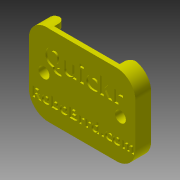
# Autodesk Inventor part: quickr_v1
Saved by Autodesk Inventor 2014 SP1 (Build 180222100, 222)
## iProperties
Created: 2014-02-28
Part Number: quickr_v1
Material: Generic
Document SubType Name: Modeling
Designer: Erin
Density: 1 g/cm^3
Appearance: Default
Author: Erin
Autodesk Inventor part; units mm, degrees
(part 1 of 3)
ref_plane "YZ Plane" through (0, 0, 0) normal (1, 0, 0) x (0, 1, 0)
ref_plane "XY Plane" through (0, 0, 0) normal (0, 0, 1) x (1, 0, 0)
sketch "Sketch1" plane through (0, 0, 0) normal (0, 1, 0) x (-1, 0, 0)
  line L0 (29.241, 31.084) -> (29.241, 17.6221)
  line L1 (0.285, 31.084) -> (0.285, 17.368)
  line L2 (4.095, 13.8121) -> (25.431, 13.8121)
  spline S0 degree 3 poles (29.241, 17.6221) (29.241, 15.518) (27.5351, 13.8121) (25.431, 13.8121) knots 0 0 0 0 1 1 1 1
  line L3 (29.241, 17.6221) -> (29.241, 15.518) construction
  line L4 (29.241, 15.518) -> (27.5351, 13.8121) construction
  line L5 (27.5351, 13.8121) -> (25.431, 13.8121) construction
  spline S1 degree 3 poles (4.095, 13.8121) (1.9909, 13.8121) (0.285, 15.518) (0.285, 17.6221) knots 0 0 0 0 1 1 1 1
  line L6 (4.095, 13.8121) -> (1.9909, 13.8121) construction
  line L7 (1.9909, 13.8121) -> (0.285, 15.518) construction
  line L8 (0.285, 15.518) -> (0.285, 17.6221) construction
  spline S2 degree 3 poles (25.431, 34.64) (27.5351, 34.64) (29.241, 32.9341) (29.241, 30.83) knots 0 0 0 0 1 1 1 1
  line L9 (25.431, 34.64) -> (27.5351, 34.64) construction
  line L10 (27.5351, 34.64) -> (29.241, 32.9341) construction
  line L11 (29.241, 32.9341) -> (29.241, 30.83) construction
  spline S3 degree 3 poles (0.285, 30.83) (0.285, 32.9341) (1.9909, 34.64) (4.095, 34.64) knots 0 0 0 0 1 1 1 1
  line L12 (0.285, 30.83) -> (0.285, 32.9341) construction
  line L13 (0.285, 32.9341) -> (1.9909, 34.64) construction
  line L14 (1.9909, 34.64) -> (4.095, 34.64) construction
  line L15 (25.431, 34.64) -> (3.841, 34.64)
  line L16 (10.9529, 29.56) -> (10.9529, 29.3061)
  spline S4 degree 3 poles (14.4582, 19.1461) (14.4582, 19.6791) (14.026, 20.1112) (13.4929, 20.1112) knots 0 0 0 0 1 1 1 1
  line L17 (14.4582, 19.1461) -> (14.4582, 19.6791) construction
  line L18 (14.4582, 19.6791) -> (14.026, 20.1112) construction
  line L19 (14.026, 20.1112) -> (13.4929, 20.1112) construction
  spline S5 degree 3 poles (13.4929, 20.1112) (12.9599, 20.1112) (12.5277, 19.6791) (12.5277, 19.1461) knots 0 0 0 0 1 1 1 1
  line L20 (13.4929, 20.1112) -> (12.9599, 20.1112) construction
  line L21 (12.9599, 20.1112) -> (12.5277, 19.6791) construction
  line L22 (12.5277, 19.6791) -> (12.5277, 19.1461) construction
  spline S6 degree 3 poles (12.5277, 19.1461) (12.5277, 18.613) (12.9599, 18.1809) (13.4929, 18.1809) knots 0 0 0 0 1 1 1 1
  line L23 (12.5277, 19.1461) -> (12.5277, 18.613) construction
  line L24 (12.5277, 18.613) -> (12.9599, 18.1809) construction
  line L25 (12.9599, 18.1809) -> (13.4929, 18.1809) construction
  spline S7 degree 3 poles (13.4929, 18.1809) (14.026, 18.1809) (14.4582, 18.613) (14.4582, 19.1461) knots 0 0 0 0 1 1 1 1
  line L26 (13.4929, 18.1809) -> (14.026, 18.1809) construction
  line L27 (14.026, 18.1809) -> (14.4582, 18.613) construction
  line L28 (14.4582, 18.613) -> (14.4582, 19.1461) construction
  spline S8 degree 3 poles (16.9982, 19.1461) (16.9982, 19.6791) (16.566, 20.1112) (16.0329, 20.1112) knots 0 0 0 0 1 1 1 1
  line L29 (16.9982, 19.1461) -> (16.9982, 19.6791) construction
  line L30 (16.9982, 19.6791) -> (16.566, 20.1112) construction
  line L31 (16.566, 20.1112) -> (16.0329, 20.1112) construction
  spline S9 degree 3 poles (16.0329, 20.1112) (15.4999, 20.1112) (15.0677, 19.6791) (15.0677, 19.1461) knots 0 0 0 0 1 1 1 1
  line L32 (16.0329, 20.1112) -> (15.4999, 20.1112) construction
  line L33 (15.4999, 20.1112) -> (15.0677, 19.6791) construction
  line L34 (15.0677, 19.6791) -> (15.0677, 19.1461) construction
  spline S10 degree 3 poles (15.0677, 19.1461) (15.0677, 18.613) (15.4999, 18.1809) (16.0329, 18.1809) knots 0 0 0 0 1 1 1 1
  line L35 (15.0677, 19.1461) -> (15.0677, 18.613) construction
  line L36 (15.0677, 18.613) -> (15.4999, 18.1809) construction
  line L37 (15.4999, 18.1809) -> (16.0329, 18.1809) construction
  spline S11 degree 3 poles (16.0329, 18.1809) (16.566, 18.1809) (16.9982, 18.613) (16.9982, 19.1461) knots 0 0 0 0 1 1 1 1
  line L38 (16.0329, 18.1809) -> (16.566, 18.1809) construction
  line L39 (16.566, 18.1809) -> (16.9982, 18.613) construction
  line L40 (16.9982, 18.613) -> (16.9982, 19.1461) construction
  spline S12 degree 3 poles (11.9182, 19.1461) (11.9182, 19.6791) (11.486, 20.1112) (10.9529, 20.1112) knots 0 0 0 0 1 1 1 1
  line L41 (11.9182, 19.1461) -> (11.9182, 19.6791) construction
  line L42 (11.9182, 19.6791) -> (11.486, 20.1112) construction
  line L43 (11.486, 20.1112) -> (10.9529, 20.1112) construction
  spline S13 degree 3 poles (10.9529, 20.1112) (10.4199, 20.1112) (9.9877, 19.6791) (9.9877, 19.1461) knots 0 0 0 0 1 1 1 1
  line L44 (10.9529, 20.1112) -> (10.4199, 20.1112) construction
  line L45 (10.4199, 20.1112) -> (9.9877, 19.6791) construction
  line L46 (9.9877, 19.6791) -> (9.9877, 19.1461) construction
  spline S14 degree 3 poles (9.9877, 19.1461) (9.9877, 18.613) (10.4199, 18.1809) (10.9529, 18.1809) knots 0 0 0 0 1 1 1 1
  line L47 (9.9877, 19.1461) -> (9.9877, 18.613) construction
  line L48 (9.9877, 18.613) -> (10.4199, 18.1809) construction
  line L49 (10.4199, 18.1809) -> (10.9529, 18.1809) construction
  spline S15 degree 3 poles (10.9529, 18.1809) (11.486, 18.1809) (11.9182, 18.613) (11.9182, 19.1461) knots 0 0 0 0 1 1 1 1
  line L50 (10.9529, 18.1809) -> (11.486, 18.1809) construction
  line L51 (11.486, 18.1809) -> (11.9182, 18.613) construction
  line L52 (11.9182, 18.613) -> (11.9182, 19.1461) construction
  spline S16 degree 3 poles (9.3782, 19.1461) (9.3782, 19.6791) (8.946, 20.1112) (8.4129, 20.1112) knots 0 0 0 0 1 1 1 1
  line L53 (9.3782, 19.1461) -> (9.3782, 19.6791) construction
  line L54 (9.3782, 19.6791) -> (8.946, 20.1112) construction
  line L55 (8.946, 20.1112) -> (8.4129, 20.1112) construction
  spline S17 degree 3 poles (8.4129, 20.1112) (7.8799, 20.1112) (7.4477, 19.6791) (7.4477, 19.1461) knots 0 0 0 0 1 1 1 1
  line L56 (8.4129, 20.1112) -> (7.8799, 20.1112) construction
  line L57 (7.8799, 20.1112) -> (7.4477, 19.6791) construction
  line L58 (7.4477, 19.6791) -> (7.4477, 19.1461) construction
  spline S18 degree 3 poles (7.4477, 19.1461) (7.4477, 18.613) (7.8799, 18.1809) (8.4129, 18.1809) knots 0 0 0 0 1 1 1 1
  line L59 (7.4477, 19.1461) -> (7.4477, 18.613) construction
  line L60 (7.4477, 18.613) -> (7.8799, 18.1809) construction
  line L61 (7.8799, 18.1809) -> (8.4129, 18.1809) construction
  spline S19 degree 3 poles (8.4129, 18.1809) (8.946, 18.1809) (9.3782, 18.613) (9.3782, 19.1461) knots 0 0 0 0 1 1 1 1
  line L62 (8.4129, 18.1809) -> (8.946, 18.1809) construction
  line L63 (8.946, 18.1809) -> (9.3782, 18.613) construction
  line L64 (9.3782, 18.613) -> (9.3782, 19.1461) construction
  spline S20 degree 3 poles (6.8382, 19.1461) (6.8382, 19.6791) (6.406, 20.1112) (5.8729, 20.1112) knots 0 0 0 0 1 1 1 1
  line L65 (6.8382, 19.1461) -> (6.8382, 19.6791) construction
  line L66 (6.8382, 19.6791) -> (6.406, 20.1112) construction
  line L67 (6.406, 20.1112) -> (5.8729, 20.1112) construction
  spline S21 degree 3 poles (5.8729, 20.1112) (5.3399, 20.1112) (4.9077, 19.6791) (4.9077, 19.1461) knots 0 0 0 0 1 1 1 1
  line L68 (5.8729, 20.1112) -> (5.3399, 20.1112) construction
  line L69 (5.3399, 20.1112) -> (4.9077, 19.6791) construction
  line L70 (4.9077, 19.6791) -> (4.9077, 19.1461) construction
  spline S22 degree 3 poles (4.9077, 19.1461) (4.9077, 18.613) (5.3399, 18.1809) (5.8729, 18.1809) knots 0 0 0 0 1 1 1 1
  line L71 (4.9077, 19.1461) -> (4.9077, 18.613) construction
  line L72 (4.9077, 18.613) -> (5.3399, 18.1809) construction
  line L73 (5.3399, 18.1809) -> (5.8729, 18.1809) construction
  spline S23 degree 3 poles (5.8729, 18.1809) (6.406, 18.1809) (6.8382, 18.613) (6.8382, 19.1461) knots 0 0 0 0 1 1 1 1
  line L74 (5.8729, 18.1809) -> (6.406, 18.1809) construction
  line L75 (6.406, 18.1809) -> (6.8382, 18.613) construction
  line L76 (6.8382, 18.613) -> (6.8382, 19.1461) construction
  spline S24 degree 3 poles (6.8382, 15.3361) (6.8382, 15.8691) (6.406, 16.3012) (5.8729, 16.3012) knots 0 0 0 0 1 1 1 1
  line L77 (6.8382, 15.3361) -> (6.8382, 15.8691) construction
  line L78 (6.8382, 15.8691) -> (6.406, 16.3012) construction
  line L79 (6.406, 16.3012) -> (5.8729, 16.3012) construction
  spline S25 degree 3 poles (5.8729, 16.3012) (5.3399, 16.3012) (4.9077, 15.8691) (4.9077, 15.3361) knots 0 0 0 0 1 1 1 1
  line L80 (5.8729, 16.3012) -> (5.3399, 16.3012) construction
  line L81 (5.3399, 16.3012) -> (4.9077, 15.8691) construction
  line L82 (4.9077, 15.8691) -> (4.9077, 15.3361) construction
  spline S26 degree 3 poles (4.9077, 15.3361) (4.9077, 14.803) (5.3399, 14.3709) (5.8729, 14.3709) knots 0 0 0 0 1 1 1 1
  line L83 (4.9077, 15.3361) -> (4.9077, 14.803) construction
  line L84 (4.9077, 14.803) -> (5.3399, 14.3709) construction
  line L85 (5.3399, 14.3709) -> (5.8729, 14.3709) construction
  spline S27 degree 3 poles (5.8729, 14.3709) (6.406, 14.3709) (6.8382, 14.803) (6.8382, 15.3361) knots 0 0 0 0 1 1 1 1
  line L86 (5.8729, 14.3709) -> (6.406, 14.3709) construction
  line L87 (6.406, 14.3709) -> (6.8382, 14.803) construction
  line L88 (6.8382, 14.803) -> (6.8382, 15.3361) construction
  spline S28 degree 3 poles (9.3782, 15.3361) (9.3782, 15.8691) (8.946, 16.3012) (8.4129, 16.3012) knots 0 0 0 0 1 1 1 1
  line L89 (9.3782, 15.3361) -> (9.3782, 15.8691) construction
  line L90 (9.3782, 15.8691) -> (8.946, 16.3012) construction
  line L91 (8.946, 16.3012) -> (8.4129, 16.3012) construction
  spline S29 degree 3 poles (8.4129, 16.3012) (7.8799, 16.3012) (7.4477, 15.8691) (7.4477, 15.3361) knots 0 0 0 0 1 1 1 1
  line L92 (8.4129, 16.3012) -> (7.8799, 16.3012) construction
  line L93 (7.8799, 16.3012) -> (7.4477, 15.8691) construction
  line L94 (7.4477, 15.8691) -> (7.4477, 15.3361) construction
  spline S30 degree 3 poles (7.4477, 15.3361) (7.4477, 14.803) (7.8799, 14.3709) (8.4129, 14.3709) knots 0 0 0 0 1 1 1 1
  line L95 (7.4477, 15.3361) -> (7.4477, 14.803) construction
  line L96 (7.4477, 14.803) -> (7.8799, 14.3709) construction
  line L97 (7.8799, 14.3709) -> (8.4129, 14.3709) construction
  spline S31 degree 3 poles (8.4129, 14.3709) (8.946, 14.3709) (9.3782, 14.803) (9.3782, 15.3361) knots 0 0 0 0 1 1 1 1
  line L98 (8.4129, 14.3709) -> (8.946, 14.3709) construction
  line L99 (8.946, 14.3709) -> (9.3782, 14.803) construction
  line L100 (9.3782, 14.803) -> (9.3782, 15.3361) construction
  spline S32 degree 3 poles (19.5382, 19.1461) (19.5382, 19.6791) (19.106, 20.1112) (18.5729, 20.1112) knots 0 0 0 0 1 1 1 1
  line L101 (19.5382, 19.1461) -> (19.5382, 19.6791) construction
  line L102 (19.5382, 19.6791) -> (19.106, 20.1112) construction
  line L103 (19.106, 20.1112) -> (18.5729, 20.1112) construction
  spline S33 degree 3 poles (18.5729, 20.1112) (18.0399, 20.1112) (17.6077, 19.6791) (17.6077, 19.1461) knots 0 0 0 0 1 1 1 1
  line L104 (18.5729, 20.1112) -> (18.0399, 20.1112) construction
  line L105 (18.0399, 20.1112) -> (17.6077, 19.6791) construction
  line L106 (17.6077, 19.6791) -> (17.6077, 19.1461) construction
  spline S34 degree 3 poles (17.6077, 19.1461) (17.6077, 18.613) (18.0399, 18.1809) (18.5729, 18.1809) knots 0 0 0 0 1 1 1 1
  line L107 (17.6077, 19.1461) -> (17.6077, 18.613) construction
  line L108 (17.6077, 18.613) -> (18.0399, 18.1809) construction
  line L109 (18.0399, 18.1809) -> (18.5729, 18.1809) construction
  spline S35 degree 3 poles (18.5729, 18.1809) (19.106, 18.1809) (19.5382, 18.613) (19.5382, 19.1461) knots 0 0 0 0 1 1 1 1
  line L110 (18.5729, 18.1809) -> (19.106, 18.1809) construction
  line L111 (19.106, 18.1809) -> (19.5382, 18.613) construction
  line L112 (19.5382, 18.613) -> (19.5382, 19.1461) construction
  spline S36 degree 3 poles (22.0782, 19.1461) (22.0782, 19.6791) (21.646, 20.1112) (21.1129, 20.1112) knots 0 0 0 0 1 1 1 1
  line L113 (22.0782, 19.1461) -> (22.0782, 19.6791) construction
  line L114 (22.0782, 19.6791) -> (21.646, 20.1112) construction
  line L115 (21.646, 20.1112) -> (21.1129, 20.1112) construction
  spline S37 degree 3 poles (21.1129, 20.1112) (20.5799, 20.1112) (20.1477, 19.6791) (20.1477, 19.1461) knots 0 0 0 0 1 1 1 1
  line L116 (21.1129, 20.1112) -> (20.5799, 20.1112) construction
  line L117 (20.5799, 20.1112) -> (20.1477, 19.6791) construction
  line L118 (20.1477, 19.6791) -> (20.1477, 19.1461) construction
  spline S38 degree 3 poles (20.1477, 19.1461) (20.1477, 18.613) (20.5799, 18.1809) (21.1129, 18.1809) knots 0 0 0 0 1 1 1 1
  line L119 (20.1477, 19.1461) -> (20.1477, 18.613) construction
  line L120 (20.1477, 18.613) -> (20.5799, 18.1809) construction
  line L121 (20.5799, 18.1809) -> (21.1129, 18.1809) construction
  spline S39 degree 3 poles (21.1129, 18.1809) (21.646, 18.1809) (22.0782, 18.613) (22.0782, 19.1461) knots 0 0 0 0 1 1 1 1
  line L122 (21.1129, 18.1809) -> (21.646, 18.1809) construction
  line L123 (21.646, 18.1809) -> (22.0782, 18.613) construction
  line L124 (22.0782, 18.613) -> (22.0782, 19.1461) construction
  spline S40 degree 3 poles (24.6182, 19.1461) (24.6182, 19.6791) (24.186, 20.1112) (23.6529, 20.1112) knots 0 0 0 0 1 1 1 1
  line L125 (24.6182, 19.1461) -> (24.6182, 19.6791) construction
  line L126 (24.6182, 19.6791) -> (24.186, 20.1112) construction
  line L127 (24.186, 20.1112) -> (23.6529, 20.1112) construction
  spline S41 degree 3 poles (23.6529, 20.1112) (23.1199, 20.1112) (22.6877, 19.6791) (22.6877, 19.1461) knots 0 0 0 0 1 1 1 1
  line L128 (23.6529, 20.1112) -> (23.1199, 20.1112) construction
  line L129 (23.1199, 20.1112) -> (22.6877, 19.6791) construction
  line L130 (22.6877, 19.6791) -> (22.6877, 19.1461) construction
  spline S42 degree 3 poles (22.6877, 19.1461) (22.6877, 18.613) (23.1199, 18.1809) (23.6529, 18.1809) knots 0 0 0 0 1 1 1 1
  line L131 (22.6877, 19.1461) -> (22.6877, 18.613) construction
  line L132 (22.6877, 18.613) -> (23.1199, 18.1809) construction
  line L133 (23.1199, 18.1809) -> (23.6529, 18.1809) construction
  spline S43 degree 3 poles (23.6529, 18.1809) (24.186, 18.1809) (24.6182, 18.613) (24.6182, 19.1461) knots 0 0 0 0 1 1 1 1
  line L134 (23.6529, 18.1809) -> (24.186, 18.1809) construction
  line L135 (24.186, 18.1809) -> (24.6182, 18.613) construction
  line L136 (24.6182, 18.613) -> (24.6182, 19.1461) construction
  spline S44 degree 3 poles (11.9182, 15.3361) (11.9182, 15.8691) (11.486, 16.3012) (10.9529, 16.3012) knots 0 0 0 0 1 1 1 1
  line L137 (11.9182, 15.3361) -> (11.9182, 15.8691) construction
  line L138 (11.9182, 15.8691) -> (11.486, 16.3012) construction
  line L139 (11.486, 16.3012) -> (10.9529, 16.3012) construction
  spline S45 degree 3 poles (10.9529, 16.3012) (10.4199, 16.3012) (9.9877, 15.8691) (9.9877, 15.3361) knots 0 0 0 0 1 1 1 1
  line L140 (10.9529, 16.3012) -> (10.4199, 16.3012) construction
  line L141 (10.4199, 16.3012) -> (9.9877, 15.8691) construction
  line L142 (9.9877, 15.8691) -> (9.9877, 15.3361) construction
  spline S46 degree 3 poles (9.9877, 15.3361) (9.9877, 14.803) (10.4199, 14.3709) (10.9529, 14.3709) knots 0 0 0 0 1 1 1 1
  line L143 (9.9877, 15.3361) -> (9.9877, 14.803) construction
  line L144 (9.9877, 14.803) -> (10.4199, 14.3709) construction
  line L145 (10.4199, 14.3709) -> (10.9529, 14.3709) construction
  spline S47 degree 3 poles (10.9529, 14.3709) (11.486, 14.3709) (11.9182, 14.803) (11.9182, 15.3361) knots 0 0 0 0 1 1 1 1
  line L146 (10.9529, 14.3709) -> (11.486, 14.3709) construction
  line L147 (11.486, 14.3709) -> (11.9182, 14.803) construction
  line L148 (11.9182, 14.803) -> (11.9182, 15.3361) construction
  spline S48 degree 3 poles (14.4582, 15.3361) (14.4582, 15.8691) (14.026, 16.3012) (13.4929, 16.3012) knots 0 0 0 0 1 1 1 1
  line L149 (14.4582, 15.3361) -> (14.4582, 15.8691) construction
  line L150 (14.4582, 15.8691) -> (14.026, 16.3012) construction
  line L151 (14.026, 16.3012) -> (13.4929, 16.3012) construction
  spline S49 degree 3 poles (13.4929, 16.3012) (12.9599, 16.3012) (12.5277, 15.8691) (12.5277, 15.3361) knots 0 0 0 0 1 1 1 1
  line L152 (13.4929, 16.3012) -> (12.9599, 16.3012) construction
  line L153 (12.9599, 16.3012) -> (12.5277, 15.8691) construction
  line L154 (12.5277, 15.8691) -> (12.5277, 15.3361) construction
  spline S50 degree 3 poles (12.5277, 15.3361) (12.5277, 14.803) (12.9599, 14.3709) (13.4929, 14.3709) knots 0 0 0 0 1 1 1 1
  line L155 (12.5277, 15.3361) -> (12.5277, 14.803) construction
  line L156 (12.5277, 14.803) -> (12.9599, 14.3709) construction
  line L157 (12.9599, 14.3709) -> (13.4929, 14.3709) construction
  spline S51 degree 3 poles (13.4929, 14.3709) (14.026, 14.3709) (14.4582, 14.803) (14.4582, 15.3361) knots 0 0 0 0 1 1 1 1
  line L158 (13.4929, 14.3709) -> (14.026, 14.3709) construction
  line L159 (14.026, 14.3709) -> (14.4582, 14.803) construction
  line L160 (14.4582, 14.803) -> (14.4582, 15.3361) construction
  spline S52 degree 3 poles (16.9982, 15.3361) (16.9982, 15.8691) (16.566, 16.3012) (16.0329, 16.3012) knots 0 0 0 0 1 1 1 1
  line L161 (16.9982, 15.3361) -> (16.9982, 15.8691) construction
  line L162 (16.9982, 15.8691) -> (16.566, 16.3012) construction
  line L163 (16.566, 16.3012) -> (16.0329, 16.3012) construction
  spline S53 degree 3 poles (16.0329, 16.3012) (15.4999, 16.3012) (15.0677, 15.8691) (15.0677, 15.3361) knots 0 0 0 0 1 1 1 1
  line L164 (16.0329, 16.3012) -> (15.4999, 16.3012) construction
  line L165 (15.4999, 16.3012) -> (15.0677, 15.8691) construction
  line L166 (15.0677, 15.8691) -> (15.0677, 15.3361) construction
  spline S54 degree 3 poles (15.0677, 15.3361) (15.0677, 14.803) (15.4999, 14.3709) (16.0329, 14.3709) knots 0 0 0 0 1 1 1 1
  line L167 (15.0677, 15.3361) -> (15.0677, 14.803) construction
  line L168 (15.0677, 14.803) -> (15.4999, 14.3709) construction
  line L169 (15.4999, 14.3709) -> (16.0329, 14.3709) construction
  spline S55 degree 3 poles (16.0329, 14.3709) (16.566, 14.3709) (16.9982, 14.803) (16.9982, 15.3361) knots 0 0 0 0 1 1 1 1
  line L170 (16.0329, 14.3709) -> (16.566, 14.3709) construction
  line L171 (16.566, 14.3709) -> (16.9982, 14.803) construction
  line L172 (16.9982, 14.803) -> (16.9982, 15.3361) construction
  spline S56 degree 3 poles (19.5382, 15.3361) (19.5382, 15.8691) (19.106, 16.3012) (18.5729, 16.3012) knots 0 0 0 0 1 1 1 1
  line L173 (19.5382, 15.3361) -> (19.5382, 15.8691) construction
  line L174 (19.5382, 15.8691) -> (19.106, 16.3012) construction
  line L175 (19.106, 16.3012) -> (18.5729, 16.3012) construction
  spline S57 degree 3 poles (18.5729, 16.3012) (18.0399, 16.3012) (17.6077, 15.8691) (17.6077, 15.3361) knots 0 0 0 0 1 1 1 1
  line L176 (18.5729, 16.3012) -> (18.0399, 16.3012) construction
  line L177 (18.0399, 16.3012) -> (17.6077, 15.8691) construction
  line L178 (17.6077, 15.8691) -> (17.6077, 15.3361) construction
  spline S58 degree 3 poles (17.6077, 15.3361) (17.6077, 14.803) (18.0399, 14.3709) (18.5729, 14.3709) knots 0 0 0 0 1 1 1 1
  line L179 (17.6077, 15.3361) -> (17.6077, 14.803) construction
  line L180 (17.6077, 14.803) -> (18.0399, 14.3709) construction
  line L181 (18.0399, 14.3709) -> (18.5729, 14.3709) construction
  spline S59 degree 3 poles (18.5729, 14.3709) (19.106, 14.3709) (19.5382, 14.803) (19.5382, 15.3361) knots 0 0 0 0 1 1 1 1
  line L182 (18.5729, 14.3709) -> (19.106, 14.3709) construction
  line L183 (19.106, 14.3709) -> (19.5382, 14.803) construction
  line L184 (19.5382, 14.803) -> (19.5382, 15.3361) construction
  spline S60 degree 3 poles (22.0782, 15.3361) (22.0782, 15.8691) (21.646, 16.3012) (21.1129, 16.3012) knots 0 0 0 0 1 1 1 1
  line L185 (22.0782, 15.3361) -> (22.0782, 15.8691) construction
  line L186 (22.0782, 15.8691) -> (21.646, 16.3012) construction
  line L187 (21.646, 16.3012) -> (21.1129, 16.3012) construction
  spline S61 degree 3 poles (21.1129, 16.3012) (20.5799, 16.3012) (20.1477, 15.8691) (20.1477, 15.3361) knots 0 0 0 0 1 1 1 1
  line L188 (21.1129, 16.3012) -> (20.5799, 16.3012) construction
  line L189 (20.5799, 16.3012) -> (20.1477, 15.8691) construction
  line L190 (20.1477, 15.8691) -> (20.1477, 15.3361) construction
  spline S62 degree 3 poles (20.1477, 15.3361) (20.1477, 14.803) (20.5799, 14.3709) (21.1129, 14.3709) knots 0 0 0 0 1 1 1 1
  line L191 (20.1477, 15.3361) -> (20.1477, 14.803) construction
  line L192 (20.1477, 14.803) -> (20.5799, 14.3709) construction
  line L193 (20.5799, 14.3709) -> (21.1129, 14.3709) construction
  spline S63 degree 3 poles (21.1129, 14.3709) (21.646, 14.3709) (22.0782, 14.803) (22.0782, 15.3361) knots 0 0 0 0 1 1 1 1
  line L194 (21.1129, 14.3709) -> (21.646, 14.3709) construction
  line L195 (21.646, 14.3709) -> (22.0782, 14.803) construction
  line L196 (22.0782, 14.803) -> (22.0782, 15.3361) construction
  spline S64 degree 3 poles (24.6182, 15.3361) (24.6182, 15.8691) (24.186, 16.3012) (23.6529, 16.3012) knots 0 0 0 0 1 1 1 1
  line L197 (24.6182, 15.3361) -> (24.6182, 15.8691) construction
  line L198 (24.6182, 15.8691) -> (24.186, 16.3012) construction
  line L199 (24.186, 16.3012) -> (23.6529, 16.3012) construction
  spline S65 degree 3 poles (23.6529, 16.3012) (23.1199, 16.3012) (22.6877, 15.8691) (22.6877, 15.3361) knots 0 0 0 0 1 1 1 1
  line L200 (23.6529, 16.3012) -> (23.1199, 16.3012) construction
  line L201 (23.1199, 16.3012) -> (22.6877, 15.8691) construction
  line L202 (22.6877, 15.8691) -> (22.6877, 15.3361) construction
  spline S66 degree 3 poles (22.6877, 15.3361) (22.6877, 14.803) (23.1199, 14.3709) (23.6529, 14.3709) knots 0 0 0 0 1 1 1 1
  line L203 (22.6877, 15.3361) -> (22.6877, 14.803) construction
  line L204 (22.6877, 14.803) -> (23.1199, 14.3709) construction
  line L205 (23.1199, 14.3709) -> (23.6529, 14.3709) construction
  spline S67 degree 3 poles (23.6529, 14.3709) (24.186, 14.3709) (24.6182, 14.803) (24.6182, 15.3361) knots 0 0 0 0 1 1 1 1
  line L206 (23.6529, 14.3709) -> (24.186, 14.3709) construction
  line L207 (24.186, 14.3709) -> (24.6182, 14.803) construction
  line L208 (24.6182, 14.803) -> (24.6182, 15.3361) construction
  spline S68 degree 3 poles (14.4582, 29.3061) (14.4582, 29.8391) (14.026, 30.2712) (13.4929, 30.2712) knots 0 0 0 0 1 1 1 1
  line L209 (14.4582, 29.3061) -> (14.4582, 29.8391) construction
  line L210 (14.4582, 29.8391) -> (14.026, 30.2712) construction
  line L211 (14.026, 30.2712) -> (13.4929, 30.2712) construction
  spline S69 degree 3 poles (13.4929, 30.2712) (12.9599, 30.2712) (12.5277, 29.8391) (12.5277, 29.3061) knots 0 0 0 0 1 1 1 1
  line L212 (13.4929, 30.2712) -> (12.9599, 30.2712) construction
  line L213 (12.9599, 30.2712) -> (12.5277, 29.8391) construction
  line L214 (12.5277, 29.8391) -> (12.5277, 29.3061) construction
  spline S70 degree 3 poles (12.5277, 29.3061) (12.5277, 28.773) (12.9599, 28.3409) (13.4929, 28.3409) knots 0 0 0 0 1 1 1 1
  line L215 (12.5277, 29.3061) -> (12.5277, 28.773) construction
  line L216 (12.5277, 28.773) -> (12.9599, 28.3409) construction
  line L217 (12.9599, 28.3409) -> (13.4929, 28.3409) construction
  spline S71 degree 3 poles (13.4929, 28.3409) (14.026, 28.3409) (14.4582, 28.773) (14.4582, 29.3061) knots 0 0 0 0 1 1 1 1
  line L218 (13.4929, 28.3409) -> (14.026, 28.3409) construction
  line L219 (14.026, 28.3409) -> (14.4582, 28.773) construction
  line L220 (14.4582, 28.773) -> (14.4582, 29.3061) construction
  spline S72 degree 3 poles (16.9982, 29.3061) (16.9982, 29.8391) (16.566, 30.2712) (16.0329, 30.2712) knots 0 0 0 0 1 1 1 1
  line L221 (16.9982, 29.3061) -> (16.9982, 29.8391) construction
  line L222 (16.9982, 29.8391) -> (16.566, 30.2712) construction
  line L223 (16.566, 30.2712) -> (16.0329, 30.2712) construction
  spline S73 degree 3 poles (16.0329, 30.2712) (15.4999, 30.2712) (15.0677, 29.8391) (15.0677, 29.3061) knots 0 0 0 0 1 1 1 1
  line L224 (16.0329, 30.2712) -> (15.4999, 30.2712) construction
  line L225 (15.4999, 30.2712) -> (15.0677, 29.8391) construction
  line L226 (15.0677, 29.8391) -> (15.0677, 29.3061) construction
  spline S74 degree 3 poles (15.0677, 29.3061) (15.0677, 28.773) (15.4999, 28.3409) (16.0329, 28.3409) knots 0 0 0 0 1 1 1 1
  line L227 (15.0677, 29.3061) -> (15.0677, 28.773) construction
  line L228 (15.0677, 28.773) -> (15.4999, 28.3409) construction
  line L229 (15.4999, 28.3409) -> (16.0329, 28.3409) construction
  spline S75 degree 3 poles (16.0329, 28.3409) (16.566, 28.3409) (16.9982, 28.773) (16.9982, 29.3061) knots 0 0 0 0 1 1 1 1
  line L230 (16.0329, 28.3409) -> (16.566, 28.3409) construction
  line L231 (16.566, 28.3409) -> (16.9982, 28.773) construction
  line L232 (16.9982, 28.773) -> (16.9982, 29.3061) construction
  spline S76 degree 3 poles (11.9182, 29.3061) (11.9182, 29.8391) (11.486, 30.2712) (10.9529, 30.2712) knots 0 0 0 0 1 1 1 1
  line L233 (11.9182, 29.3061) -> (11.9182, 29.8391) construction
  line L234 (11.9182, 29.8391) -> (11.486, 30.2712) construction
  line L235 (11.486, 30.2712) -> (10.9529, 30.2712) construction
  spline S77 degree 3 poles (10.9529, 30.2712) (10.4199, 30.2712) (9.9877, 29.8391) (9.9877, 29.3061) knots 0 0 0 0 1 1 1 1
  line L236 (10.9529, 30.2712) -> (10.4199, 30.2712) construction
  line L237 (10.4199, 30.2712) -> (9.9877, 29.8391) construction
  line L238 (9.9877, 29.8391) -> (9.9877, 29.3061) construction
  spline S78 degree 3 poles (9.9877, 29.3061) (9.9877, 28.773) (10.4199, 28.3409) (10.9529, 28.3409) knots 0 0 0 0 1 1 1 1
  line L239 (9.9877, 29.3061) -> (9.9877, 28.773) construction
  line L240 (9.9877, 28.773) -> (10.4199, 28.3409) construction
  line L241 (10.4199, 28.3409) -> (10.9529, 28.3409) construction
  spline S79 degree 3 poles (10.9529, 28.3409) (11.486, 28.3409) (11.9182, 28.773) (11.9182, 29.3061) knots 0 0 0 0 1 1 1 1
  line L242 (10.9529, 28.3409) -> (11.486, 28.3409) construction
  line L243 (11.486, 28.3409) -> (11.9182, 28.773) construction
  line L244 (11.9182, 28.773) -> (11.9182, 29.3061) construction
  spline S80 degree 3 poles (19.5382, 29.3061) (19.5382, 29.8391) (19.106, 30.2712) (18.5729, 30.2712) knots 0 0 0 0 1 1 1 1
  line L245 (19.5382, 29.3061) -> (19.5382, 29.8391) construction
  line L246 (19.5382, 29.8391) -> (19.106, 30.2712) construction
  line L247 (19.106, 30.2712) -> (18.5729, 30.2712) construction
  spline S81 degree 3 poles (18.5729, 30.2712) (18.0399, 30.2712) (17.6077, 29.8391) (17.6077, 29.3061) knots 0 0 0 0 1 1 1 1
  line L248 (18.5729, 30.2712) -> (18.0399, 30.2712) construction
  line L249 (18.0399, 30.2712) -> (17.6077, 29.8391) construction
  line L250 (17.6077, 29.8391) -> (17.6077, 29.3061) construction
  spline S82 degree 3 poles (17.6077, 29.3061) (17.6077, 28.773) (18.0399, 28.3409) (18.5729, 28.3409) knots 0 0 0 0 1 1 1 1
  line L251 (17.6077, 29.3061) -> (17.6077, 28.773) construction
  line L252 (17.6077, 28.773) -> (18.0399, 28.3409) construction
  line L253 (18.0399, 28.3409) -> (18.5729, 28.3409) construction
  spline S83 degree 3 poles (18.5729, 28.3409) (19.106, 28.3409) (19.5382, 28.773) (19.5382, 29.3061) knots 0 0 0 0 1 1 1 1
  line L254 (18.5729, 28.3409) -> (19.106, 28.3409) construction
  line L255 (19.106, 28.3409) -> (19.5382, 28.773) construction
  line L256 (19.5382, 28.773) -> (19.5382, 29.3061) construction
  spline S84 degree 3 poles (22.0782, 29.3061) (22.0782, 29.8391) (21.646, 30.2712) (21.1129, 30.2712) knots 0 0 0 0 1 1 1 1
  line L257 (22.0782, 29.3061) -> (22.0782, 29.8391) construction
  line L258 (22.0782, 29.8391) -> (21.646, 30.2712) construction
  line L259 (21.646, 30.2712) -> (21.1129, 30.2712) construction
  spline S85 degree 3 poles (21.1129, 30.2712) (20.5799, 30.2712) (20.1477, 29.8391) (20.1477, 29.3061) knots 0 0 0 0 1 1 1 1
  line L260 (21.1129, 30.2712) -> (20.5799, 30.2712) construction
  line L261 (20.5799, 30.2712) -> (20.1477, 29.8391) construction
  line L262 (20.1477, 29.8391) -> (20.1477, 29.3061) construction
  spline S86 degree 3 poles (20.1477, 29.3061) (20.1477, 28.773) (20.5799, 28.3409) (21.1129, 28.3409) knots 0 0 0 0 1 1 1 1
  line L263 (20.1477, 29.3061) -> (20.1477, 28.773) construction
  line L264 (20.1477, 28.773) -> (20.5799, 28.3409) construction
  line L265 (20.5799, 28.3409) -> (21.1129, 28.3409) construction
  spline S87 degree 3 poles (21.1129, 28.3409) (21.646, 28.3409) (22.0782, 28.773) (22.0782, 29.3061) knots 0 0 0 0 1 1 1 1
  line L266 (21.1129, 28.3409) -> (21.646, 28.3409) construction
  line L267 (21.646, 28.3409) -> (22.0782, 28.773) construction
  line L268 (22.0782, 28.773) -> (22.0782, 29.3061) construction
  spline S88 degree 3 poles (24.6182, 29.3061) (24.6182, 29.8391) (24.186, 30.2712) (23.6529, 30.2712) knots 0 0 0 0 1 1 1 1
  line L269 (24.6182, 29.3061) -> (24.6182, 29.8391) construction
  line L270 (24.6182, 29.8391) -> (24.186, 30.2712) construction
  line L271 (24.186, 30.2712) -> (23.6529, 30.2712) construction
  spline S89 degree 3 poles (23.6529, 30.2712) (23.1199, 30.2712) (22.6877, 29.8391) (22.6877, 29.3061) knots 0 0 0 0 1 1 1 1
  line L272 (23.6529, 30.2712) -> (23.1199, 30.2712) construction
  line L273 (23.1199, 30.2712) -> (22.6877, 29.8391) construction
  line L274 (22.6877, 29.8391) -> (22.6877, 29.3061) construction
  spline S90 degree 3 poles (22.6877, 29.3061) (22.6877, 28.773) (23.1199, 28.3409) (23.6529, 28.3409) knots 0 0 0 0 1 1 1 1
  line L275 (22.6877, 29.3061) -> (22.6877, 28.773) construction
  line L276 (22.6877, 28.773) -> (23.1199, 28.3409) construction
  line L277 (23.1199, 28.3409) -> (23.6529, 28.3409) construction
  spline S91 degree 3 poles (23.6529, 28.3409) (24.186, 28.3409) (24.6182, 28.773) (24.6182, 29.3061) knots 0 0 0 0 1 1 1 1
  line L278 (23.6529, 28.3409) -> (24.186, 28.3409) construction
  line L279 (24.186, 28.3409) -> (24.6182, 28.773) construction
  line L280 (24.6182, 28.773) -> (24.6182, 29.3061) construction
  spline S92 degree 3 poles (9.3782, 29.3061) (9.3782, 29.8391) (8.946, 30.2712) (8.4129, 30.2712) knots 0 0 0 0 1 1 1 1
  line L281 (9.3782, 29.3061) -> (9.3782, 29.8391) construction
  line L282 (9.3782, 29.8391) -> (8.946, 30.2712) construction
  line L283 (8.946, 30.2712) -> (8.4129, 30.2712) construction
  spline S93 degree 3 poles (8.4129, 30.2712) (7.8799, 30.2712) (7.4477, 29.8391) (7.4477, 29.3061) knots 0 0 0 0 1 1 1 1
  line L284 (8.4129, 30.2712) -> (7.8799, 30.2712) construction
  line L285 (7.8799, 30.2712) -> (7.4477, 29.8391) construction
  line L286 (7.4477, 29.8391) -> (7.4477, 29.3061) construction
  spline S94 degree 3 poles (7.4477, 29.3061) (7.4477, 28.773) (7.8799, 28.3409) (8.4129, 28.3409) knots 0 0 0 0 1 1 1 1
  line L287 (7.4477, 29.3061) -> (7.4477, 28.773) construction
  line L288 (7.4477, 28.773) -> (7.8799, 28.3409) construction
  line L289 (7.8799, 28.3409) -> (8.4129, 28.3409) construction
  spline S95 degree 3 poles (8.4129, 28.3409) (8.946, 28.3409) (9.3782, 28.773) (9.3782, 29.3061) knots 0 0 0 0 1 1 1 1
  line L290 (8.4129, 28.3409) -> (8.946, 28.3409) construction
  line L291 (8.946, 28.3409) -> (9.3782, 28.773) construction
  line L292 (9.3782, 28.773) -> (9.3782, 29.3061) construction
  spline S96 degree 3 poles (6.8382, 29.3061) (6.8382, 29.8391) (6.406, 30.2712) (5.8729, 30.2712) knots 0 0 0 0 1 1 1 1
  line L293 (6.8382, 29.3061) -> (6.8382, 29.8391) construction
  line L294 (6.8382, 29.8391) -> (6.406, 30.2712) construction
  line L295 (6.406, 30.2712) -> (5.8729, 30.2712) construction
  spline S97 degree 3 poles (5.8729, 30.2712) (5.3399, 30.2712) (4.9077, 29.8391) (4.9077, 29.3061) knots 0 0 0 0 1 1 1 1
  line L296 (5.8729, 30.2712) -> (5.3399, 30.2712) construction
  line L297 (5.3399, 30.2712) -> (4.9077, 29.8391) construction
  line L298 (4.9077, 29.8391) -> (4.9077, 29.3061) construction
  spline S98 degree 3 poles (4.9077, 29.3061) (4.9077, 28.773) (5.3399, 28.3409) (5.8729, 28.3409) knots 0 0 0 0 1 1 1 1
  line L299 (4.9077, 29.3061) -> (4.9077, 28.773) construction
  line L300 (4.9077, 28.773) -> (5.3399, 28.3409) construction
  line L301 (5.3399, 28.3409) -> (5.8729, 28.3409) construction
  spline S99 degree 3 poles (5.8729, 28.3409) (6.406, 28.3409) (6.8382, 28.773) (6.8382, 29.3061) knots 0 0 0 0 1 1 1 1
  line L302 (5.8729, 28.3409) -> (6.406, 28.3409) construction
  line L303 (6.406, 28.3409) -> (6.8382, 28.773) construction
  line L304 (6.8382, 28.773) -> (6.8382, 29.3061) construction
  spline S100 degree 3 poles (6.8382, 33.1161) (6.8382, 33.6491) (6.406, 34.0812) (5.8729, 34.0812) knots 0 0 0 0 1 1 1 1
  line L305 (6.8382, 33.1161) -> (6.8382, 33.6491) construction
  line L306 (6.8382, 33.6491) -> (6.406, 34.0812) construction
  line L307 (6.406, 34.0812) -> (5.8729, 34.0812) construction
  spline S101 degree 3 poles (5.8729, 34.0812) (5.3399, 34.0812) (4.9077, 33.6491) (4.9077, 33.1161) knots 0 0 0 0 1 1 1 1
  line L308 (5.8729, 34.0812) -> (5.3399, 34.0812) construction
  line L309 (5.3399, 34.0812) -> (4.9077, 33.6491) construction
  line L310 (4.9077, 33.6491) -> (4.9077, 33.1161) construction
  spline S102 degree 3 poles (4.9077, 33.1161) (4.9077, 32.583) (5.3399, 32.1509) (5.8729, 32.1509) knots 0 0 0 0 1 1 1 1
  line L311 (4.9077, 33.1161) -> (4.9077, 32.583) construction
  line L312 (4.9077, 32.583) -> (5.3399, 32.1509) construction
  line L313 (5.3399, 32.1509) -> (5.8729, 32.1509) construction
  spline S103 degree 3 poles (5.8729, 32.1509) (6.406, 32.1509) (6.8382, 32.583) (6.8382, 33.1161) knots 0 0 0 0 1 1 1 1
  line L314 (5.8729, 32.1509) -> (6.406, 32.1509) construction
  line L315 (6.406, 32.1509) -> (6.8382, 32.583) construction
  line L316 (6.8382, 32.583) -> (6.8382, 33.1161) construction
  spline S104 degree 3 poles (9.3782, 33.1161) (9.3782, 33.6491) (8.946, 34.0812) (8.4129, 34.0812) knots 0 0 0 0 1 1 1 1
  line L317 (9.3782, 33.1161) -> (9.3782, 33.6491) construction
  line L318 (9.3782, 33.6491) -> (8.946, 34.0812) construction
  line L319 (8.946, 34.0812) -> (8.4129, 34.0812) construction
  spline S105 degree 3 poles (8.4129, 34.0812) (7.8799, 34.0812) (7.4477, 33.6491) (7.4477, 33.1161) knots 0 0 0 0 1 1 1 1
  line L320 (8.4129, 34.0812) -> (7.8799, 34.0812) construction
  line L321 (7.8799, 34.0812) -> (7.4477, 33.6491) construction
  line L322 (7.4477, 33.6491) -> (7.4477, 33.1161) construction
  spline S106 degree 3 poles (7.4477, 33.1161) (7.4477, 32.583) (7.8799, 32.1509) (8.4129, 32.1509) knots 0 0 0 0 1 1 1 1
  line L323 (7.4477, 33.1161) -> (7.4477, 32.583) construction
  line L324 (7.4477, 32.583) -> (7.8799, 32.1509) construction
  line L325 (7.8799, 32.1509) -> (8.4129, 32.1509) construction
  spline S107 degree 3 poles (8.4129, 32.1509) (8.946, 32.1509) (9.3782, 32.583) (9.3782, 33.1161) knots 0 0 0 0 1 1 1 1
  line L326 (8.4129, 32.1509) -> (8.946, 32.1509) construction
  line L327 (8.946, 32.1509) -> (9.3782, 32.583) construction
  line L328 (9.3782, 32.583) -> (9.3782, 33.1161) construction
  spline S108 degree 3 poles (11.9182, 33.1161) (11.9182, 33.6491) (11.486, 34.0812) (10.9529, 34.0812) knots 0 0 0 0 1 1 1 1
  line L329 (11.9182, 33.1161) -> (11.9182, 33.6491) construction
  line L330 (11.9182, 33.6491) -> (11.486, 34.0812) construction
  line L331 (11.486, 34.0812) -> (10.9529, 34.0812) construction
  spline S109 degree 3 poles (10.9529, 34.0812) (10.4199, 34.0812) (9.9877, 33.6491) (9.9877, 33.1161) knots 0 0 0 0 1 1 1 1
  line L332 (10.9529, 34.0812) -> (10.4199, 34.0812) construction
  line L333 (10.4199, 34.0812) -> (9.9877, 33.6491) construction
  line L334 (9.9877, 33.6491) -> (9.9877, 33.1161) construction
  spline S110 degree 3 poles (9.9877, 33.1161) (9.9877, 32.583) (10.4199, 32.1509) (10.9529, 32.1509) knots 0 0 0 0 1 1 1 1
  line L335 (9.9877, 33.1161) -> (9.9877, 32.583) construction
  line L336 (9.9877, 32.583) -> (10.4199, 32.1509) construction
  line L337 (10.4199, 32.1509) -> (10.9529, 32.1509) construction
  spline S111 degree 3 poles (10.9529, 32.1509) (11.486, 32.1509) (11.9182, 32.583) (11.9182, 33.1161) knots 0 0 0 0 1 1 1 1
  line L338 (10.9529, 32.1509) -> (11.486, 32.1509) construction
  line L339 (11.486, 32.1509) -> (11.9182, 32.583) construction
  line L340 (11.9182, 32.583) -> (11.9182, 33.1161) construction
  spline S112 degree 3 poles (16.9982, 33.1161) (16.9982, 33.6491) (16.566, 34.0812) (16.0329, 34.0812) knots 0 0 0 0 1 1 1 1
  line L341 (16.9982, 33.1161) -> (16.9982, 33.6491) construction
  line L342 (16.9982, 33.6491) -> (16.566, 34.0812) construction
  line L343 (16.566, 34.0812) -> (16.0329, 34.0812) construction
  spline S113 degree 3 poles (16.0329, 34.0812) (15.4999, 34.0812) (15.0677, 33.6491) (15.0677, 33.1161) knots 0 0 0 0 1 1 1 1
  line L344 (16.0329, 34.0812) -> (15.4999, 34.0812) construction
  line L345 (15.4999, 34.0812) -> (15.0677, 33.6491) construction
  line L346 (15.0677, 33.6491) -> (15.0677, 33.1161) construction
  spline S114 degree 3 poles (15.0677, 33.1161) (15.0677, 32.583) (15.4999, 32.1509) (16.0329, 32.1509) knots 0 0 0 0 1 1 1 1
  line L347 (15.0677, 33.1161) -> (15.0677, 32.583) construction
  line L348 (15.0677, 32.583) -> (15.4999, 32.1509) construction
  line L349 (15.4999, 32.1509) -> (16.0329, 32.1509) construction
  spline S115 degree 3 poles (16.0329, 32.1509) (16.566, 32.1509) (16.9982, 32.583) (16.9982, 33.1161) knots 0 0 0 0 1 1 1 1
  line L350 (16.0329, 32.1509) -> (16.566, 32.1509) construction
  line L351 (16.566, 32.1509) -> (16.9982, 32.583) construction
  line L352 (16.9982, 32.583) -> (16.9982, 33.1161) construction
  spline S116 degree 3 poles (19.5382, 33.1161) (19.5382, 33.6491) (19.106, 34.0812) (18.5729, 34.0812) knots 0 0 0 0 1 1 1 1
  line L353 (19.5382, 33.1161) -> (19.5382, 33.6491) construction
  line L354 (19.5382, 33.6491) -> (19.106, 34.0812) construction
  line L355 (19.106, 34.0812) -> (18.5729, 34.0812) construction
  spline S117 degree 3 poles (18.5729, 34.0812) (18.0399, 34.0812) (17.6077, 33.6491) (17.6077, 33.1161) knots 0 0 0 0 1 1 1 1
  line L356 (18.5729, 34.0812) -> (18.0399, 34.0812) construction
  line L357 (18.0399, 34.0812) -> (17.6077, 33.6491) construction
  line L358 (17.6077, 33.6491) -> (17.6077, 33.1161) construction
  spline S118 degree 3 poles (17.6077, 33.1161) (17.6077, 32.583) (18.0399, 32.1509) (18.5729, 32.1509) knots 0 0 0 0 1 1 1 1
  line L359 (17.6077, 33.1161) -> (17.6077, 32.583) construction
  line L360 (17.6077, 32.583) -> (18.0399, 32.1509) construction
  line L361 (18.0399, 32.1509) -> (18.5729, 32.1509) construction
  spline S119 degree 3 poles (18.5729, 32.1509) (19.106, 32.1509) (19.5382, 32.583) (19.5382, 33.1161) knots 0 0 0 0 1 1 1 1
  line L362 (18.5729, 32.1509) -> (19.106, 32.1509) construction
  line L363 (19.106, 32.1509) -> (19.5382, 32.583) construction
  line L364 (19.5382, 32.583) -> (19.5382, 33.1161) construction
  spline S120 degree 3 poles (22.0782, 33.1161) (22.0782, 33.6491) (21.646, 34.0812) (21.1129, 34.0812) knots 0 0 0 0 1 1 1 1
  line L365 (22.0782, 33.1161) -> (22.0782, 33.6491) construction
  line L366 (22.0782, 33.6491) -> (21.646, 34.0812) construction
  line L367 (21.646, 34.0812) -> (21.1129, 34.0812) construction
  spline S121 degree 3 poles (21.1129, 34.0812) (20.5799, 34.0812) (20.1477, 33.6491) (20.1477, 33.1161) knots 0 0 0 0 1 1 1 1
  line L368 (21.1129, 34.0812) -> (20.5799, 34.0812) construction
  line L369 (20.5799, 34.0812) -> (20.1477, 33.6491) construction
  line L370 (20.1477, 33.6491) -> (20.1477, 33.1161) construction
  spline S122 degree 3 poles (20.1477, 33.1161) (20.1477, 32.583) (20.5799, 32.1509) (21.1129, 32.1509) knots 0 0 0 0 1 1 1 1
  line L371 (20.1477, 33.1161) -> (20.1477, 32.583) construction
  line L372 (20.1477, 32.583) -> (20.5799, 32.1509) construction
  line L373 (20.5799, 32.1509) -> (21.1129, 32.1509) construction
  spline S123 degree 3 poles (21.1129, 32.1509) (21.646, 32.1509) (22.0782, 32.583) (22.0782, 33.1161) knots 0 0 0 0 1 1 1 1
  line L374 (21.1129, 32.1509) -> (21.646, 32.1509) construction
  line L375 (21.646, 32.1509) -> (22.0782, 32.583) construction
  line L376 (22.0782, 32.583) -> (22.0782, 33.1161) construction
  spline S124 degree 3 poles (24.6182, 33.1161) (24.6182, 33.6491) (24.186, 34.0812) (23.6529, 34.0812) knots 0 0 0 0 1 1 1 1
  line L377 (24.6182, 33.1161) -> (24.6182, 33.6491) construction
  line L378 (24.6182, 33.6491) -> (24.186, 34.0812) construction
  line L379 (24.186, 34.0812) -> (23.6529, 34.0812) construction
  spline S125 degree 3 poles (23.6529, 34.0812) (23.1199, 34.0812) (22.6877, 33.6491) (22.6877, 33.1161) knots 0 0 0 0 1 1 1 1
  line L380 (23.6529, 34.0812) -> (23.1199, 34.0812) construction
  line L381 (23.1199, 34.0812) -> (22.6877, 33.6491) construction
  line L382 (22.6877, 33.6491) -> (22.6877, 33.1161) construction
  spline S126 degree 3 poles (22.6877, 33.1161) (22.6877, 32.583) (23.1199, 32.1509) (23.6529, 32.1509) knots 0 0 0 0 1 1 1 1
  line L383 (22.6877, 33.1161) -> (22.6877, 32.583) construction
  line L384 (22.6877, 32.583) -> (23.1199, 32.1509) construction
  line L385 (23.1199, 32.1509) -> (23.6529, 32.1509) construction
  spline S127 degree 3 poles (23.6529, 32.1509) (24.186, 32.1509) (24.6182, 32.583) (24.6182, 33.1161) knots 0 0 0 0 1 1 1 1
  line L386 (23.6529, 32.1509) -> (24.186, 32.1509) construction
  line L387 (24.186, 32.1509) -> (24.6182, 32.583) construction
  line L388 (24.6182, 32.583) -> (24.6182, 33.1161) construction
  spline S128 degree 3 poles (14.4582, 33.1161) (14.4582, 33.6491) (14.026, 34.0812) (13.4929, 34.0812) knots 0 0 0 0 1 1 1 1
  line L389 (14.4582, 33.1161) -> (14.4582, 33.6491) construction
  line L390 (14.4582, 33.6491) -> (14.026, 34.0812) construction
  line L391 (14.026, 34.0812) -> (13.4929, 34.0812) construction
  spline S129 degree 3 poles (13.4929, 34.0812) (12.9599, 34.0812) (12.5277, 33.6491) (12.5277, 33.1161) knots 0 0 0 0 1 1 1 1
  line L392 (13.4929, 34.0812) -> (12.9599, 34.0812) construction
  line L393 (12.9599, 34.0812) -> (12.5277, 33.6491) construction
  line L394 (12.5277, 33.6491) -> (12.5277, 33.1161) construction
  spline S130 degree 3 poles (12.5277, 33.1161) (12.5277, 32.583) (12.9599, 32.1509) (13.4929, 32.1509) knots 0 0 0 0 1 1 1 1
  line L395 (12.5277, 33.1161) -> (12.5277, 32.583) construction
  line L396 (12.5277, 32.583) -> (12.9599, 32.1509) construction
  line L397 (12.9599, 32.1509) -> (13.4929, 32.1509) construction
  spline S131 degree 3 poles (13.4929, 32.1509) (14.026, 32.1509) (14.4582, 32.583) (14.4582, 33.1161) knots 0 0 0 0 1 1 1 1
  line L398 (13.4929, 32.1509) -> (14.026, 32.1509) construction
  line L399 (14.026, 32.1509) -> (14.4582, 32.583) construction
  line L400 (14.4582, 32.583) -> (14.4582, 33.1161) construction
  spline S132 degree 3 poles (3.7648, 24.2261) (3.7648, 24.8853) (3.2303, 25.4198) (2.571, 25.4198) knots 0 0 0 0 1 1 1 1
  line L401 (3.7648, 24.2261) -> (3.7648, 24.8853) construction
  line L402 (3.7648, 24.8853) -> (3.2303, 25.4198) construction
  line L403 (3.2303, 25.4198) -> (2.571, 25.4198) construction
  spline S133 degree 3 poles (2.571, 25.4198) (1.9118, 25.4198) (1.3772, 24.8853) (1.3772, 24.2261) knots 0 0 0 0 1 1 1 1
  line L404 (2.571, 25.4198) -> (1.9118, 25.4198) construction
  line L405 (1.9118, 25.4198) -> (1.3772, 24.8853) construction
  line L406 (1.3772, 24.8853) -> (1.3772, 24.2261) construction
  spline S134 degree 3 poles (1.3772, 24.2261) (1.3772, 23.5668) (1.9118, 23.0323) (2.571, 23.0323) knots 0 0 0 0 1 1 1 1
  line L407 (1.3772, 24.2261) -> (1.3772, 23.5668) construction
  line L408 (1.3772, 23.5668) -> (1.9118, 23.0323) construction
  line L409 (1.9118, 23.0323) -> (2.571, 23.0323) construction
  spline S135 degree 3 poles (2.571, 23.0323) (3.2303, 23.0323) (3.7648, 23.5668) (3.7648, 24.2261) knots 0 0 0 0 1 1 1 1
  line L410 (2.571, 23.0323) -> (3.2303, 23.0323) construction
  line L411 (3.2303, 23.0323) -> (3.7648, 23.5668) construction
  line L412 (3.7648, 23.5668) -> (3.7648, 24.2261) construction
  spline S136 degree 3 poles (28.1488, 24.2261) (28.1488, 24.8853) (27.6142, 25.4198) (26.955, 25.4198) knots 0 0 0 0 1 1 1 1
  line L413 (28.1488, 24.2261) -> (28.1488, 24.8853) construction
  line L414 (28.1488, 24.8853) -> (27.6142, 25.4198) construction
  line L415 (27.6142, 25.4198) -> (26.955, 25.4198) construction
  spline S137 degree 3 poles (26.955, 25.4198) (26.2957, 25.4198) (25.7612, 24.8853) (25.7612, 24.2261) knots 0 0 0 0 1 1 1 1
  line L416 (26.955, 25.4198) -> (26.2957, 25.4198) construction
  line L417 (26.2957, 25.4198) -> (25.7612, 24.8853) construction
  line L418 (25.7612, 24.8853) -> (25.7612, 24.2261) construction
  spline S138 degree 3 poles (25.7612, 24.2261) (25.7612, 23.5668) (26.2957, 23.0323) (26.955, 23.0323) knots 0 0 0 0 1 1 1 1
  line L419 (25.7612, 24.2261) -> (25.7612, 23.5668) construction
  line L420 (25.7612, 23.5668) -> (26.2957, 23.0323) construction
  line L421 (26.2957, 23.0323) -> (26.955, 23.0323) construction
  spline S139 degree 3 poles (26.955, 23.0323) (27.6142, 23.0323) (28.1488, 23.5668) (28.1488, 24.2261) knots 0 0 0 0 1 1 1 1
  line L422 (26.955, 23.0323) -> (27.6142, 23.0323) construction
  line L423 (27.6142, 23.0323) -> (28.1488, 23.5668) construction
  line L424 (28.1488, 23.5668) -> (28.1488, 24.2261) construction
  spline S140 degree 3 poles (3.7139, 24.2261) (3.7139, 24.8572) (3.2021, 25.369) (2.571, 25.369) knots 0 0 0 0 1 1 1 1
  line L425 (3.7139, 24.2261) -> (3.7139, 24.8572) construction
  line L426 (3.7139, 24.8572) -> (3.2021, 25.369) construction
  line L427 (3.2021, 25.369) -> (2.571, 25.369) construction
  spline S141 degree 3 poles (2.571, 25.369) (1.9399, 25.369) (1.4279, 24.8572) (1.4279, 24.2261) knots 0 0 0 0 1 1 1 1
  line L428 (2.571, 25.369) -> (1.9399, 25.369) construction
  line L429 (1.9399, 25.369) -> (1.4279, 24.8572) construction
  line L430 (1.4279, 24.8572) -> (1.4279, 24.2261) construction
  spline S142 degree 3 poles (1.4279, 24.2261) (1.4279, 23.5949) (1.9399, 23.083) (2.571, 23.083) knots 0 0 0 0 1 1 1 1
  line L431 (1.4279, 24.2261) -> (1.4279, 23.5949) construction
  line L432 (1.4279, 23.5949) -> (1.9399, 23.083) construction
  line L433 (1.9399, 23.083) -> (2.571, 23.083) construction
  spline S143 degree 3 poles (2.571, 23.083) (3.2021, 23.083) (3.7139, 23.5949) (3.7139, 24.2261) knots 0 0 0 0 1 1 1 1
  line L434 (2.571, 23.083) -> (3.2021, 23.083) construction
  line L435 (3.2021, 23.083) -> (3.7139, 23.5949) construction
  line L436 (3.7139, 23.5949) -> (3.7139, 24.2261) construction
  spline S144 degree 3 poles (28.0979, 24.2261) (28.0979, 24.8572) (27.5861, 25.369) (26.955, 25.369) knots 0 0 0 0 1 1 1 1
  line L437 (28.0979, 24.2261) -> (28.0979, 24.8572) construction
  line L438 (28.0979, 24.8572) -> (27.5861, 25.369) construction
  line L439 (27.5861, 25.369) -> (26.955, 25.369) construction
  spline S145 degree 3 poles (26.955, 25.369) (26.3239, 25.369) (25.812, 24.8572) (25.812, 24.2261) knots 0 0 0 0 1 1 1 1
  line L440 (26.955, 25.369) -> (26.3239, 25.369) construction
  line L441 (26.3239, 25.369) -> (25.812, 24.8572) construction
  line L442 (25.812, 24.8572) -> (25.812, 24.2261) construction
  spline S146 degree 3 poles (25.812, 24.2261) (25.812, 23.5949) (26.3239, 23.083) (26.955, 23.083) knots 0 0 0 0 1 1 1 1
  line L443 (25.812, 24.2261) -> (25.812, 23.5949) construction
  line L444 (25.812, 23.5949) -> (26.3239, 23.083) construction
  line L445 (26.3239, 23.083) -> (26.955, 23.083) construction
  spline S147 degree 3 poles (26.955, 23.083) (27.5861, 23.083) (28.0979, 23.5949) (28.0979, 24.2261) knots 0 0 0 0 1 1 1 1
  line L446 (26.955, 23.083) -> (27.5861, 23.083) construction
  line L447 (27.5861, 23.083) -> (28.0979, 23.5949) construction
  line L448 (28.0979, 23.5949) -> (28.0979, 24.2261) construction
  spline S148 degree 3 poles (13.9375, 19.1461) (13.9375, 19.3915) (13.7384, 19.5905) (13.4929, 19.5905) knots 0 0 0 0 1 1 1 1
  line L449 (13.9375, 19.1461) -> (13.9375, 19.3915) construction
  line L450 (13.9375, 19.3915) -> (13.7384, 19.5905) construction
  line L451 (13.7384, 19.5905) -> (13.4929, 19.5905) construction
  spline S149 degree 3 poles (13.4929, 19.5905) (13.2475, 19.5905) (13.0485, 19.3915) (13.0485, 19.1461) knots 0 0 0 0 1 1 1 1
  line L452 (13.4929, 19.5905) -> (13.2475, 19.5905) construction
  line L453 (13.2475, 19.5905) -> (13.0485, 19.3915) construction
  line L454 (13.0485, 19.3915) -> (13.0485, 19.1461) construction
  spline S150 degree 3 poles (13.0485, 19.1461) (13.0485, 18.9006) (13.2475, 18.7015) (13.4929, 18.7015) knots 0 0 0 0 1 1 1 1
  line L455 (13.0485, 19.1461) -> (13.0485, 18.9006) construction
  line L456 (13.0485, 18.9006) -> (13.2475, 18.7015) construction
  line L457 (13.2475, 18.7015) -> (13.4929, 18.7015) construction
  spline S151 degree 3 poles (13.4929, 18.7015) (13.7384, 18.7015) (13.9375, 18.9006) (13.9375, 19.1461) knots 0 0 0 0 1 1 1 1
  line L458 (13.4929, 18.7015) -> (13.7384, 18.7015) construction
  line L459 (13.7384, 18.7015) -> (13.9375, 18.9006) construction
  line L460 (13.9375, 18.9006) -> (13.9375, 19.1461) construction
  spline S152 degree 3 poles (16.4775, 19.1461) (16.4775, 19.3915) (16.2784, 19.5905) (16.0329, 19.5905) knots 0 0 0 0 1 1 1 1
  line L461 (16.4775, 19.1461) -> (16.4775, 19.3915) construction
  line L462 (16.4775, 19.3915) -> (16.2784, 19.5905) construction
  line L463 (16.2784, 19.5905) -> (16.0329, 19.5905) construction
  spline S153 degree 3 poles (16.0329, 19.5905) (15.7875, 19.5905) (15.5885, 19.3915) (15.5885, 19.1461) knots 0 0 0 0 1 1 1 1
  line L464 (16.0329, 19.5905) -> (15.7875, 19.5905) construction
  line L465 (15.7875, 19.5905) -> (15.5885, 19.3915) construction
  line L466 (15.5885, 19.3915) -> (15.5885, 19.1461) construction
  spline S154 degree 3 poles (15.5885, 19.1461) (15.5885, 18.9006) (15.7875, 18.7015) (16.0329, 18.7015) knots 0 0 0 0 1 1 1 1
  line L467 (15.5885, 19.1461) -> (15.5885, 18.9006) construction
  line L468 (15.5885, 18.9006) -> (15.7875, 18.7015) construction